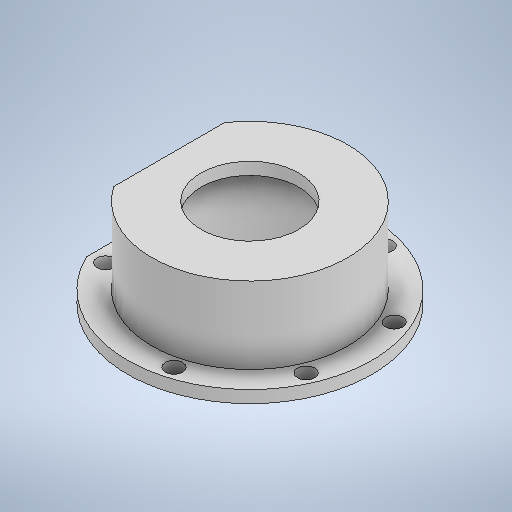
# Autodesk Inventor part: B1 fixe2
Saved by Autodesk Inventor 2025 (Build 290162000, 162)
## iProperties
Created: 2025-01-16
Part Number: B1 fixe2
Material: Générique
Document SubType Name: Modeling
Designer: adrie
Density: 1 g/cm^3
Appearance: Par défaut
Author: adrie
Autodesk Inventor part; units mm, degrees
ref_plane "YZ Plane" through (0, 0, 0) normal (1, 0, 0) x (0, 1, 0)
ref_plane "XZ Plane" through (0, 0, 0) normal (0, 1, 0) x (-1, 0, 0)
ref_plane "XY Plane" through (0, 0, 0) normal (0, 0, 1) x (1, 0, 0)
sketch "Esquisse1" plane through (0, 0, 0) normal (0, 1, 0) x (-1, 0, 0)
  circle A0 centre (0, 0) radius 31
  circle A1 centre (0, 0) radius 50
  circle A2 centre (0, 0) radius 40
  line L0 (45, -21.7945) -> (45, 21.7945)
  dimension "d0" = 62
  dimension "d1" = 100
  dimension "d2" = 80
  dimension "d47" = 45
  constraints: 3 centre point, 3 coincident, 2 end point, 2 point on circle, 1 vertical
  measures "d0" diameter of A0
  measures "d1" diameter of A1
  measures "d2" diameter of A2
  measures "d47" distance from line of L0 point (0, 0)
extrude "Extrusion1" add sketch "Esquisse1" along normal blind 5 contours A1 L0 | L0 A1 | A2
sketch "Esquisse2" plane through (0, 5, 0) normal (0, 1, 0) x (1, 0, 0)
  circle A0 centre (0, 0) radius 40
  circle A1 centre (0, 0) radius 31 projected
  circle A2 centre (0, 0) radius 31
  dimension "d6" = 80
  dimension "d75" = 0
  constraints: 2 centre point, 2 coincident
  measures "d6" diameter of A0
  measures "d75" radial gap between concentric circles of A2 A1
extrude "Extrusion2" add sketch "Esquisse2" along normal blind 26.3
sketch "Esquisse3" plane through (0, 31.3, 0) normal (0, 1, 0) x (1, 0, 0)
  circle A0 centre (0, 0) radius 20
  circle A1 centre (0, 0) radius 40
  circle A2 centre (0, 0) radius 40 projected
  dimension "d9" = 40
  dimension "d63" = 0
  constraints: 2 centre point, 2 coincident
  measures "d9" diameter of A0
  measures "d63" radial gap between concentric circles of A2 A1
extrude "Extrusion3" add sketch "Esquisse3" along normal blind 5
sketch "Esquisse5" plane through (0, 36.3, 0) normal (0, 1, 0) x (1, 0, 0)
  line L0 (-33, 22.6053) -> (-33, -22.6053)
  circle A0 centre (0, 0) radius 40
  circle A1 centre (0, 0) radius 40 projected
  point P0 (-33, 22.6053)
  dimension "d71" = 80
  dimension "d72" = 33
  constraints: 2 end point, 2 point on circle, 1 centre point, 1 coincident, 1 vertical
  measures "d71" diameter of A0
  measures "d72" distance from line of L0 point (0, 0)
extrude "Extrusion4" cut sketch "Esquisse5" against normal up to surface (31.3 mm away) contours L0 A0 picked at (-34.2788, -5.1971)
sketch "Esquisse6" plane through (0, 5, 0) normal (0, 1, 0) x (1, 0, 0)
  point P0 (0, 0)
sketch "Esquisse7" plane through (0, 5, 0) normal (0, 1, 0) x (1, 0, 0)
  line L0 (12, 65.0926) -> (12, -68.5298) construction
  circle A0 centre (0, 0) radius 20 construction
  circle A1 centre (12, 43) radius 3.5
  circle A2 centre (12, -43) radius 3.5
  point P0 (-37.5, -12.5)
  point P1 (-37.5, 12.5)
  dimension "d53" = 12
  dimension "d54" = 7
  dimension "d55" = 7
  dimension "d56" = 43
  dimension "d57" = 43
  constraints: 2 centre point, 2 end point, 2 point on line, 1 vertical
  measures "d53" distance from line of A0.centre L0
  measures "d54" diameter of A2
  measures "d55" diameter of A1
  measures "d56" vertical distance of A0.centre A1.centre
  measures "d57" vertical distance of A0.centre A2.centre
extrude "Extrusion6" cut sketch "Esquisse7" against normal blind 10
sketch "Esquisse8" plane through (0, 5, 0) normal (0, 1, 0) x (1, 0, 0)
  line L0 (-45, 21.7945) -> (-45, -21.7945)
  circle A0 centre (0, 0) radius 50
  dimension "d73" = 45
  dimension "d74" = 100
  constraints: 2 end point, 2 point on circle, 1 centre point, 1 coincident, 1 vertical
  measures "d73" distance from line of L0 point (0, 0)
  measures "d74" diameter of A0
extrude "Extrusion7" cut sketch "Esquisse8" against normal blind 5 contours L0 A0 picked at (-46.0601, 4.4554)
sketch "Esquisse9" plane through (0, 5, 0) normal (0, 1, 0) x (1, 0, 0)
  line L0 (41, 168.1574) -> (41, -90.4051) construction
  circle A0 centre (41, 18) radius 3.5
  circle A1 centre (41, -18) radius 3.5
  circle A2 centre (0, 0) radius 20 projected
  dimension "d58" = 7
  dimension "d59" = 7
  dimension "d60" = 18
  dimension "d61" = 18
  dimension "d62" = 41
  constraints: 2 centre point, 2 end point, 2 point on line, 1 vertical
  measures "d58" diameter of A1
  measures "d59" diameter of A0
  measures "d60" vertical distance of A2.centre A0.centre
  measures "d61" vertical distance of A2.centre A1.centre
  measures "d62" distance from line of L0 A2.centre
extrude "Extrusion8" cut sketch "Esquisse9" against normal blind 5 contours A0 | A1
sketch "Sketch10" plane through (0, 0, 0) normal (0, -1, 0) x (1, 0, 0)
  line L0 (-39, -54.8136) -> (-39, 70.7566) construction
  circle A0 centre (-39, -20) radius 3.5
  circle A1 centre (-39, 20) radius 3.5
  point P0 (0, 0)
  dimension "d64" = 39
  dimension "d65" = 20
  dimension "d66" = 20
  dimension "d67" = 7
  dimension "d68" = 7
  constraints: 2 centre point, 2 end point, 2 point on line, 1 vertical
  measures "d64" distance from line of L0 point (0, 0)
  measures "d65" vertical distance of point (0, 0) A0.centre
  measures "d66" vertical distance of A1.centre point (0, 0)
  measures "d67" diameter of A0
  measures "d68" diameter of A1
extrude "Extrusion9" cut sketch "Sketch10" against normal blind 5
equation "\"d55\" = d54"
equation "\"d57\" = d56"
equation "\"d59\" = d58"
equation "\"d61\" = d60"
equation "\"d68\" = d67"
